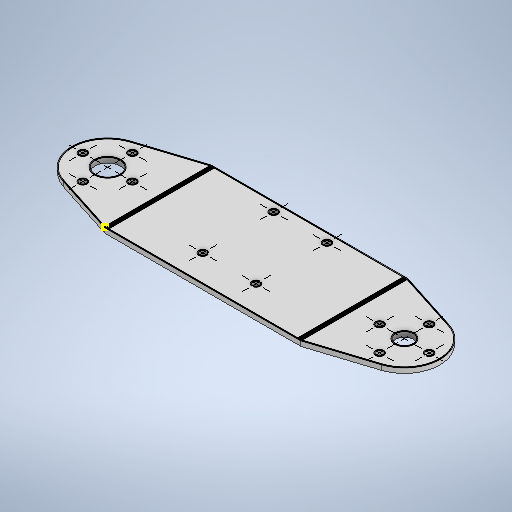
# Autodesk Inventor part: axis_19_bottom_frame
Saved by Autodesk Inventor 2025.2 (Build 292293000, 293)
## iProperties
Created: 2025-08-12
Part Number: axis_19_bottom_frame
Material: Generic
Document SubType Name: Modeling
Designer: LG
Density: 1 g/cm^3
Appearance: Default
Author: LG
Autodesk Inventor part; units mm, degrees
ref_plane "YZ Plane" through (0, 0, 0) normal (1, 0, 0) x (0, 1, 0)
ref_plane "XZ Plane" through (0, 0, 0) normal (0, 1, 0) x (-1, 0, 0)
ref_plane "XY Plane" through (0, 0, 0) normal (0, 0, 1) x (1, 0, 0)
sketch "Sketch1" plane through (0, 0, 0) normal (0, 1, 0) x (-1, 0, 0)
  line L0 (-0.4496, -30) -> (-0.4496, 0)
  line L1 (-54.9089, 0) -> (-54.9089, -30)
  circle A0 centre (-20.1543, -27.5) radius 1.05
  circle A1 centre (-20.1543, -7.5) radius 1.05
  circle A2 centre (-35.2043, -27.5) radius 1.05
  circle A3 centre (-35.2043, -7.5) radius 1.05
  circle A4 centre (-69.5486, -15) radius 2.6
  circle A5 centre (14.19, -15) radius 3.6
  circle A6 centre (7.19, -15) radius 1.05
  circle A7 centre (14.19, -22) radius 1.05
  circle A8 centre (21.19, -15) radius 1.05
  circle A9 centre (14.19, -8) radius 1.05
  circle A10 centre (-69.5486, -22) radius 1.05
  circle A11 centre (-62.5486, -15) radius 1.05
  circle A12 centre (-69.5486, -8) radius 1.05
  circle A13 centre (-76.5486, -15) radius 1.05
  line L2 (-72.585, -24.4859) -> (-55.3586, -30)
  line L3 (0, -30) -> (17.2264, -24.4859)
  arc A14 (-72.585, -5.5141) -> (-72.585, -24.4859) centre (-69.5486, -15) ccw
  arc A15 (17.2264, -24.4859) -> (17.2264, -5.5141) centre (14.19, -15) ccw
  line L4 (-55.3586, 0) -> (-72.585, -5.5141)
  line L5 (17.2264, -5.5141) -> (0, 0)
  line L6 (-55.3586, 0) -> (0, 0)
  line L7 (0, -30) -> (-55.3586, -30)
  line L8 (-55.3586, -30) -> (-55.3586, 0)
  line L9 (-54.4593, 0) -> (-54.4593, -30)
  line L10 (-0.8993, -30) -> (-0.8993, 0)
  line L11 (0, 0) -> (0, -30)
  constraints: 24 end point, 16 centre point, 12 equal radius, 8 point on line, 7 parallel, 6 vertical, 4 point on circle, 4 tangent, 2 horizontal, 2 perpendicular, 51 other
extrude "Extrusion1" add sketch "Sketch1" against normal blind 1.5
body "Solid1"
